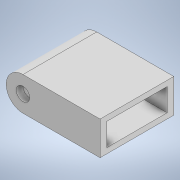
# Autodesk Inventor part: 2nd arm
Saved by Autodesk Inventor 2022 (Build 260153000, 153)
## iProperties
Created: 2021-06-29
Part Number: 2nd arm
Material: Generic
Document SubType Name: Modeling
Designer: USER
Density: 1 g/cm^3
Appearance: Default
Author: USER
Autodesk Inventor part; units mm, degrees
ref_plane "YZ Plane" through (0, 0, 0) normal (1, 0, 0) x (0, 1, 0)
ref_plane "XZ Plane" through (0, 0, 0) normal (0, 1, 0) x (-1, 0, 0)
ref_plane "XY Plane" through (0, 0, 0) normal (0, 0, 1) x (1, 0, 0)
sketch "Sketch1" plane through (0, 0, 0) normal (0, 0, 1) x (1, 0, 0)
  line L0 (-40, 12.5) -> (40, 12.5)
  line L1 (40, 12.5) -> (40, -12.5)
  line L2 (40, -12.5) -> (-40, -12.5)
  line L3 (-40, -12.5) -> (-40, 12.5)
  line L4 (-40, 12.5) -> (40, -12.5) construction
  line L5 (40, 12.5) -> (-40, -12.5) construction
  point P0 (0, 0)
  dimension "d0" = 80
  dimension "d1" = 25
  constraints: 12 end point, 2 midpoint, 2 parallel, 1 horizontal, 1 perpendicular
  measures "d0" distance of L1.end L2.end
  measures "d1" distance of L0.end L1.end
extrude "Extrusion1" add sketch "Sketch1" along normal blind 55
sketch "Sketch2" plane through (0, 0, 55) normal (0, 0, 1) x (1, 0, 0)
  circle A0 centre (-27.5, 0) radius 5
  line L0 (-40, 12.5) -> (-40, -12.5) projected
  point P0 (0, 0)
  dimension "d4" = 10
  dimension "d5" = 12.5
  constraints: 1 centre point
  measures "d4" diameter of A0
  measures "d5" distance from line of L0 A0.centre
extrude "Extrusion2" cut sketch "Sketch2" against normal through all
sketch "Sketch3" plane through (40, -12.5, 0) normal (1, 0, 0) x (0, 0, -1)
  line L0 (-50, 4) -> (-5, 4)
  line L1 (-5, 4) -> (-5, 21)
  line L2 (-5, 21) -> (-50, 21)
  line L3 (-50, 21) -> (-50, 4)
  line L4 (-50, 4) -> (-5, 21) construction
  line L5 (-5, 4) -> (-50, 21) construction
  line L6 (-55, 0) -> (-55, 25) projected
  line L7 (0, 25) -> (-55, 25) projected
  point P0 (0, 12.5)
  point P1 (-27.5, 12.5)
  dimension "d8" = 45
  dimension "d9" = 17
  dimension "d10" = 27.5
  dimension "d11" = 12.5
  constraints: 12 end point, 2 midpoint, 2 parallel, 1 horizontal, 1 perpendicular
  measures "d8" distance of L2.end L1.end
  measures "d9" distance of L1.end L0.end
  measures "d10" distance from line of L6 point (-27.5, 12.5)
  measures "d11" distance from line of L7 point (-27.5, 12.5)
extrude "Extrusion3" cut sketch "Sketch3" against normal blind 73.25
full round fillet "Full Round Fillet1" first side at (15.5833, 8.5, 20) centre faces at (-33.25, -2.8333, 20) second side at (15.5833, -8.5, 35)
fillet "Fillet1" radius 12.5 2 edges at (-40, 12.5, 27.5) (-40, -12.5, 27.5)
sketch "Sketch4" plane through (40, -12.5, 0) normal (1, 0, 0) x (0, 0, -1)
  line L0 (-55, 0) -> (-55, 25) projected
  line L1 (0, 0) -> (-55, 0) projected
  line L2 (-55, 25) -> (0, 25)
  line L3 (0, 25) -> (0, 0)
  line L4 (0, 0) -> (-55, 0)
  line L5 (-55, 0) -> (-55, 25)
  point P0 (0, 12.5)
  constraints: 8 end point, 2 parallel, 1 horizontal, 1 perpendicular
extrude "Extrusion4" cut sketch "Sketch4" against normal blind 10
body "Solid1"
